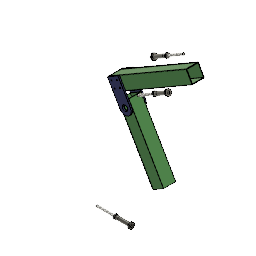
Kerbecs (Autodesk Fusion 360 design; units mm, degrees)
Autodesk Fusion 360 part; units mm, degrees
cylinder "CylinderPrimitive3" add diameter 18 height 736 placed x (0, 0, -1) y (0, 1, 0) z (1, 0, 0) at (0, 0, 0) makes body 1
copy_body "CopyPasteBodies4" bodies 1 makes body 2
move_body "Move2" bodies 2 to x (1, 0, 0) y (0, 1, 0) z (0, 0, 1) at (0, 218, 0)
copy_body "CopyPasteBodies5" bodies 1 2 makes body 3 makes body 4
move_body "Move3" bodies 3 to x (1, 0, 0) y (0, 1, 0) z (0, 0, 1) at (0, 79, 0)
move_body "Move4" bodies 4 to x (1, 0, 0) y (0, 1, 0) z (0, 0, 1) at (0, -79, 0)
cylinder "CylinderPrimitive4" add diameter 18 height 436 placed x (1, 0, 0) y (0, 0, -1) z (0, 1, 0) at (0, 0, 25) separate body makes body 5
move_body "Move5" bodies 5 to x (1, 0, 0) y (0, 1, 0) z (0, 0, 1) at (0, -109, 0)
move_body "Move6" bodies 5 to x (1, 0, 0) y (0, 1, 0) z (0, 0, 1) at (0, 0, -7)
move_body "Move7" bodies 5 to x (1, 0, 0) y (0, 1, 0) z (0, 0, 1) at (9, 0, 0)
copy_body "CopyPasteBodies6" bodies 5 makes body 6
move_body "Move8" bodies 6 to x (1, 0, 0) y (0, 1, 0) z (0, 0, 1) at (318, 0, 0)
copy_body "CopyPasteBodies7" bodies 6 makes body 7
move_body "Move9" bodies 7 to x (1, 0, 0) y (0, 1, 0) z (0, 0, 1) at (132, 0, 0)
copy_body "CopyPasteBodies8" bodies 7 makes body 8
move_body "Move10" bodies 8 to x (1, 0, 0) y (0, 1, 0) z (0, 0, 1) at (318, 0, 0)
move_face "OffsetFaces1" offset 50 1 faces at (736, 0.3267, 5.1676) on bodies 1
move_face "OffsetFaces2" offset 50 1 faces at (736, 79.3267, 5.1676) on bodies 3
move_face "OffsetFaces3" offset 50 1 faces at (736, 141.3455, -1.8705) on bodies 4
move_face "OffsetFaces4" offset 50 1 faces at (736, 220.3455, -1.8705) on bodies 2
move_body "Move11" bodies 5 to x (1, 0, 0) y (0, 1, 0) z (0, 0, 1) at (-18, 0, 0)
move_body "Move12" bodies 5 to x (1, 0, 0) y (0, 1, 0) z (0, 0, 1) at (0, 0, -18)
move_body "Move13" bodies 8 to x (1, 0, 0) y (0, 1, 0) z (0, 0, 1) at (18, 0, -18)
move_body "Move14" bodies 6 7 to x (1, 0, 0) y (0, 1, 0) z (0, 0, 1) at (0, 0, -36)
cylinder "CylinderPrimitive5" add diameter 18 height 200 placed x (1, 0, 0) y (0, 0, -1) z (0, 1, 0) at (0, 0, -75) separate body makes body 9
move_body "Move16" bodies 9 to x (1, 0, 0) y (0, 1, 0) z (0, 0, 1) at (0, -500, 0)
move_body "Move17" bodies 9 to x (1, 0, 0) y (0, 1, 0) z (0, 0, 1) at (0, 0, 75)
move_body "Move18" bodies 9 to x (1, 0, 0) y (0, 0.573576, 0.819152) z (0, -0.819152, 0.573576) at (0, -220.5842, 405.7382)
copy_body "CopyPasteBodies10" bodies 9 makes body 10
move_body "Move19" bodies 10 to x (1, 0, 0) y (0, 1, 0) z (0, 0, 1) at (75, 0, 0)
move_body "Move20" bodies 9 to x (1, 0, 0) y (0, 0.573576, -0.819152) z (0, 0.819152, 0.573576) at (0, -212.1269, -425.492)
move_body "Move21" bodies 10 to x (1, 0, 0) y (0, 0.573576, -0.819152) z (0, 0.819152, 0.573576) at (0, -212.1269, -425.492)
sketch "Sketch8" plane through (0, -506.2875, 0) normal (0, -1, 0) x (1, 0, 0)
  circle A0 centre (0, -12.0782) radius 9
  circle A1 centre (0, -12.0782) radius 9
  line L0 (-13.0767, -7.0782) -> (-23.0767, -7.0782)
  line L1 (-23.0767, -7.0782) -> (-23.0767, -11.0782)
  line L2 (-23.0767, -11.0782) -> (-13.9642, -11.0782)
  line L3 (-13.0767, -17.0782) -> (-23.0767, -17.0782)
  line L4 (-23.0767, -17.0782) -> (-23.0767, -13.0782)
  line L5 (-23.0767, -13.0782) -> (-13.9642, -13.0782)
  arc A2 (-13.0767, -17.0782) -> (13.0767, -17.0782) centre (0, -12.0782) ccw
  arc A3 (13.0767, -7.0782) -> (-13.0767, -7.0782) centre (0, -12.0782) ccw
  line L6 (13.0767, -7.0782) -> (37.5, -7.0782)
  line L7 (13.0767, -17.0782) -> (37.5, -17.0782)
  line L8 (-13.9642, -11.0782) -> (-8.9443, -11.0782)
  line L9 (-13.9642, -13.0782) -> (-8.9443, -13.0782)
  line L10 (98.0767, -11.0782) -> (88.9642, -11.0782)
  line L11 (98.0767, -17.0782) -> (98.0767, -13.0782)
  line L12 (88.0767, -17.0782) -> (98.0767, -17.0782)
  circle A4 centre (75, -12.0782) radius 9
  line L13 (98.0767, -13.0782) -> (88.9642, -13.0782)
  line L14 (61.9233, -17.0782) -> (37.5, -17.0782)
  line L15 (61.9233, -7.0782) -> (37.5, -7.0782)
  arc A5 (88.0767, -7.0782) -> (61.9233, -7.0782) centre (75, -12.0782) ccw
  line L16 (88.0767, -7.0782) -> (98.0767, -7.0782)
  line L17 (88.9642, -13.0782) -> (83.9443, -13.0782)
  arc A6 (61.9233, -17.0782) -> (88.0767, -17.0782) centre (75, -12.0782) ccw
  line L18 (88.9642, -11.0782) -> (83.9443, -11.0782)
  circle A7 centre (75, -12.0782) radius 9
  line L19 (98.0767, -7.0782) -> (98.0767, -11.0782)
  point P0 (75, 0)
  dimension "d85" = 18
  dimension "d86" = 28
  dimension "d90" = 10
  dimension "d91" = 4
  dimension "d92" = 4
  constraint concentric A0 A1
  constraint concentric A1 A2
  constraint coincident A3.start A2
  constraint horizontal L0
  constraint perpendicular L0 L1
  constraint perpendicular L1 L2
  constraint perpendicular L1 L3
  constraint perpendicular L3 L4
  constraint perpendicular L4 L5
  constraint concentric A2 A3
  constraint coincident A1 L8.end
  constraint parallel L2 L8
  constraint coincident A1 L9.end
  constraint parallel L5 L9
  measures "d85" diameter of A1
  measures "d86" diameter of A2
  measures "d90" distance of L0.start L0.end
  measures "d91" distance of L0.end L1.end
  measures "d92" distance of L3.end L4.end
extrude "Extrude4" add sketch "Sketch8" along normal blind 30 separate body contours A0 A1 L0 L1 L2 L3 L4 L5 A2 A3 L6 L7 L8 L9 L10 L11 L12 A4 L13 L14 L15 A5 L16 L17 A6 L18 A7 L19 makes body 11
move_body "Move23" bodies 11 to x (1, 0, 0) y (0, 1, 0) z (0, 0, 1) at (0, -35, 0)
copy_body "CopyPasteBodies11" bodies 11 makes body 12
move_body "Move24" bodies 12 to x (1, 0, 0) y (0, 1, 0) z (0, 0, 1) at (0, -60, 0)
move_body "Move25" bodies 11 to x (1, 0, 0) y (0, 1, 0) z (0, 0, 1) at (0, 230, 0)
move_body "Move26" bodies 12 to x (1, 0, 0) y (0, 1, 0) z (0, 0, 1) at (0, 130, 0)
box "BoxPrimitive1" add length 10 width 215 height 285 placed x (0, 1, 0) y (-1, 0, 0) z (0, 0, 1) at (215, 0, 0) separate body makes body 13
box "BoxPrimitive7" add length 44.45 width 44.45 height 250 placed x (0, 1, 0) y (-1, 0, 0) z (0, 0, 1) at (44.45, 0, 0) separate body makes body 14 in component "Shin"
move_body "Move3'" bodies 14 to x (0.866025, 0, 0.5) y (0, 1, 0) z (-0.5, 0, 0.866025) at (0, 0, 0) in component "Shin"
sketch "Sketch8 (2)" plane through (0, 0, 0) normal (0, -1, 0) x (1, 0, 0) in component "Shin"
  line L0 (-125, 216.5064) -> (0, 0)
  line L1 (0, 0) -> (38.4948, 22.225)
  line L2 (38.4948, 22.225) -> (-86.5052, 238.7314)
  line L3 (-86.5052, 238.7314) -> (-125, 216.5064)
  line L4 (-125, 216.5064) -> (-113.8875, 197.2589)
  line L5 (-113.8875, 197.2589) -> (-94.6401, 208.3714)
  circle A0 centre (-94.6401, 208.3714) radius 9.5
  dimension "d190" = 22.225
  dimension "d191" = 22.225
  dimension "d192" = 19
  constraint coincident L0.start L3.end
  constraint perpendicular L3 L4
  constraint perpendicular L2 L5
  constraint coincident L5.end A0.centre
  measures "d190" distance of L0.start L4.end
  measures "d191" distance of L4.end L5.end
  measures "d192" diameter of A0
hole "Hole1" at (-94.6401, 0, 208.3714) direction (0, 1, 0) diameter 19 depth 44.45 tip angle 180 bodies 14 in component "Shin"
shell "Shell1" thickness 2 removed faces 0 bodies 14 in component "Shin"
sketch "Sketch9" plane through (0, 0, 0) normal (0, -1, 0) x (1, 0, 0) in component "Shin"
  circle A0 centre (-94.6401, 208.3714) radius 9.5
  line L0 (-125, 216.5064) -> (0, 0)
  line L1 (0, 0) -> (38.4948, 22.225)
  line L2 (38.4948, 22.225) -> (-86.5052, 238.7314)
  line L3 (-125, 216.5064) -> (-113.8875, 197.2589)
  line L4 (-75.3927, 219.4839) -> (-86.5052, 238.7314)
  arc A1 (-113.8875, 197.2589) -> (-75.3927, 219.4839) centre (-94.6401, 208.3714) ccw
  line L5 (-125, 216.5064) -> (-149.725, 259.3313)
  line L6 (-86.5052, 238.7314) -> (-111.2302, 281.5563)
  line L7 (-149.725, 259.3313) -> (-111.2302, 281.5563)
  dimension "d199" = 49.45
  constraint coincident L0.start L3.start
  constraint coincident L2.end L4.end
  constraint tangent L3 A1
  constraint tangent L4 A1
  constraint coincident L0 L3.end
  constraint coincident L2 L4.start
  constraint parallel L5 L6
  constraint perpendicular L6 L7
  measures "d199" distance of L0.start L5.end
extrude "Extrude1" add sketch "Sketch9" along normal blind 5 separate body contours L0 L2 L3 L4 A1 L5 L6 L7 makes body 15 in component "Shin"
sketch "Sketch10" plane through (0, -5, 0) normal (0, -1, 0) x (1, 0, 0) in component "Shin"
  circle A0 centre (-94.6401, 208.3714) radius 9.5
  line L0 (-149.725, 259.3313) -> (-113.8875, 197.2589)
  arc A1 (-113.8875, 197.2589) -> (-75.3927, 219.4839) centre (-94.6401, 208.3714) ccw
  line L1 (-75.3927, 219.4839) -> (-111.2302, 281.5563)
  line L2 (-111.2302, 281.5563) -> (-149.725, 259.3313)
  line L3 (-149.725, 259.3313) -> (-144.1687, 249.7076)
  line L4 (-144.1687, 249.7076) -> (-134.545, 255.2638)
  circle A2 centre (-134.545, 255.2638) radius 2
  line L5 (-149.725, 259.3313) -> (-130.4776, 270.4438)
  line L6 (-130.4776, 270.4438) -> (-124.9213, 260.8201)
  line L7 (-149.725, 259.3313) -> (-138.6125, 240.0839)
  line L8 (-138.6125, 240.0839) -> (-100.1177, 262.3089)
  circle A3 centre (-115.2976, 266.3763) radius 2
  circle A4 centre (-123.4325, 236.0164) radius 2
  circle A5 centre (-104.1851, 247.1289) radius 2
  dimension "d206" = 11.1125
  dimension "d207" = 11.1125
  dimension "d208" = 4
  dimension "d212" = 22.225
  constraint coincident L0.start L2.end
  constraint perpendicular L2 L3
  constraint perpendicular L0 L4
  constraint coincident L4.end A2.centre
  constraint midpoint L2 L5.end
  constraint perpendicular L4 L6
  constraint perpendicular L4 L7
  constraint coincident L1 L8.end
  constraint perpendicular L1 L8
  constraint symmetric A2 L6 A3
  constraint symmetric A2 L8 A4
  constraint symmetric L8 A3 A5
  measures "d206" distance of L0.start L3.end
  measures "d207" distance of L3.end L4.end
  measures "d208" diameter of A2
  measures "d212" distance of L0.start L7.end
hole "Hole3" at (-134.545, -5, 255.2638) direction (0, 1, 0) diameter 4 depth 5 tip angle 180 bodies 15 in component "Shin"
hole "Hole2" at (-134.545, -5, 255.2638) direction (0, 1, 0) diameter 4 depth 5 tip angle 180 bodies 15 in component "Shin"
hole "Hole4" at (-115.2976, -5, 266.3763) direction (0, 1, 0) diameter 4 depth 5 tip angle 180 bodies 15 in component "Shin"
hole "Hole5" at (-123.4325, -5, 236.0164) direction (0, 1, 0) diameter 4 depth 5 tip angle 180 bodies 15 in component "Shin"
hole "Hole6" at (-104.1851, -5, 247.1289) direction (0, 1, 0) diameter 4 depth 5 tip angle 180 bodies 15 in component "Shin"
ref_plane "WorkPlane4" through (-109.3509, 22.225, 233.8514) normal (0, 1, 0) x (-1, 0, 0) in component "Shin"
mirror "Mirror1" about plane through (-109.3509, 22.225, 233.8514) normal (0, 1, 0) of bodies 15 makes body 16 in component "Shin"
sketch "Sketch11" plane through (0, 0, 0) normal (0.5, 0, -0.866025) x (0, 1, 0) in component "Shin"
  line L0 (44.45, 0) -> (44.45, 44.45)
  line L1 (44.45, 44.45) -> (0, 44.45)
  line L2 (0, 44.45) -> (0, 0)
  line L3 (0, 0) -> (44.45, 0)
  line L4 (2, 2) -> (42.45, 2)
  line L5 (42.45, 2) -> (42.45, 42.45)
  line L6 (42.45, 42.45) -> (2, 42.45)
  line L7 (2, 42.45) -> (2, 2)
  dimension "d227" = -2
extrude "Extrude2" cut sketch "Sketch11" against normal through all contours L4 L5 L6 L7 bodies 14 in component "Shin"
ref_plane "WorkPlane3" through (-149.725, 44.45, 259.3313) normal (0.866025, 0, 0.5) x (0, 1, 0) in component "Thigh"
sketch "Sketch2" plane through (-149.725, 44.45, 259.3313) normal (0.866025, 0, 0.5) x (0, 1, 0) in component "Thigh"
  line L0 (0, 0) -> (-44.45, 0)
  line L1 (0, 0) -> (0, -44.45)
  dimension "d230" = 44.45
  dimension "d231" = 44.45
  constraint coincident L0.start L1.start
  constraint horizontal L0
  constraint perpendicular L0 L1
  measures "d230" distance of L0.start L0.end
  measures "d231" distance of L0.start L1.end
box "BoxPrimitive1'" add length 44.45 width 44.45 height 320 placed x (0.5, 0, -0.866025) y (0, 1, 0) z (0.866025, 0, 0.5) at (-149.725, 0, 259.3313) separate body makes body 17 in component "Thigh"
sketch "Sketch3" plane through (0, 0, 0) normal (0, -1, 0) x (1, 0, 0) in component "Thigh"
  line L0 (127.4031, 419.3313) -> (-149.725, 259.3313)
  line L1 (-149.725, 259.3313) -> (-127.5, 220.8365)
  line L2 (-127.5, 220.8365) -> (149.6281, 380.8365)
  line L3 (149.6281, 380.8365) -> (127.4031, 419.3313)
  line L4 (-149.725, 259.3313) -> (-144.1687, 249.7076)
  line L5 (-144.1687, 249.7076) -> (-134.545, 255.2638)
  circle A0 centre (-134.545, 255.2638) radius 2
  line L6 (-149.725, 259.3313) -> (-138.6125, 240.0839)
  line L7 (-138.6125, 240.0839) -> (-119.3651, 251.1964)
  line L8 (-119.3651, 251.1964) -> (-130.4776, 270.4438)
  circle A1 centre (-115.2976, 266.3763) radius 2
  circle A2 centre (-104.1851, 247.1289) radius 2
  circle A3 centre (-123.4325, 236.0164) radius 2
  dimension "d237" = 11.1125
  dimension "d238" = 11.1125
  dimension "d239" = 4
  dimension "d241" = 22.225
  dimension "d242" = 22.225
  dimension "d243" = 22.225
  constraint coincident L0.end L1.start
  constraint perpendicular L0 L4
  constraint perpendicular L1 L5
  constraint coincident L5.end A0.centre
  constraint perpendicular L5 L6
  constraint perpendicular L1 L7
  constraint perpendicular L7 L8
  constraint symmetric A0 L8 A1
  constraint symmetric A0 L7 A3
  constraint symmetric L7 A1 A2
  measures "d237" distance of L0.end L4.end
  measures "d238" distance of L4.end L5.end
  measures "d239" diameter of A0
  measures "d241" distance of L0.end L6.end
  measures "d242" distance of L6.end L7.end
  measures "d243" distance of L7.end L8.end
shell "Shell1'" thickness 2 removed faces 1 at (-142.3167, 29.6333, 246.4997) on bodies 17 in component "Thigh"
hole "Hole1'" at (-134.545, 0, 255.2638) direction (0, 1, 0) diameter 4 depth 44.45 tip angle 180 bodies 17 in component "Thigh"
hole "Hole2'" at (-115.2976, 0, 266.3763) direction (0, 1, 0) diameter 4 depth 44.45 tip angle 180 bodies 17 in component "Thigh"
hole "Hole3'" at (-123.4325, 0, 236.0164) direction (0, 1, 0) diameter 4 depth 44.45 tip angle 180 bodies 17 in component "Thigh"
hole "Hole4'" at (-104.1851, 0, 247.1289) direction (0, 1, 0) diameter 4 depth 44.45 tip angle 180 bodies 17 in component "Thigh"
delete_face "DeleteFace1" 1 faces at (133.4127, 28.9667, 404.9223) on bodies 17 in component "Thigh"
move_face "OffsetFaces1'" offset 17.225 2 faces at (-136.8934, -1.6667, 266.7396) (-136.8934, 46.1167, 266.7396) on bodies 15 16 in component "Shin"
move_face "MoveFace1" to x (1, 0, 0) y (0, 1, 0) z (0, 0, 1) at (-8.6125, 0, 14.9173) 8 faces at (-115.9817, -3.3333, 264.497) (-135.0386, -3.3333, 257.202) (-104.8692, -3.3333, 245.2496) (-124.1166, -3.3333, 234.1371) (-115.9817, 47.7833, 268.2557) (-134.0515, 47.7833, 257.202) (-124.1166, 47.7833, 237.8958) (-104.8692, 47.7833, 249.0083) on bodies 15 16 in component "Shin"
copy_body "Body->Comp1" bodies 14 removing the originals makes body 18 in component "Bone"
copy_body "Body->Comp2" bodies 16 removing the originals makes body 19 in component "Component"
copy_body "Body->Comp3" bodies 15 removing the originals makes body 20 in component "Component'"
cylinder "CylinderPrimitive1" add diameter 8 height 100 placed x (0, 0, -1) y (0, 1, 0) z (1, 0, 0) at (0, -200, 50) separate body makes body 21 in component "Component''"
thread "Thread1" "ISO Metric profile 8.0 M8x1.25 6g" major diameter 7.866 minor diameter 6.4455 pitch 1.25 angle 60 resizes the face on face at (33.3333, -198.087, 53.5129) on bodies 21 in component "Component''"
cylinder "CylinderPrimitive1'" add diameter 15 height 5 placed x (0, 0, -1) y (0, 1, 0) z (1, 0, 0) at (100, -200, 50) separate body makes body 22 in component "Component'''"
hole "Hole1''" at (105, -200, 50) direction (-1, 0, 0) diameter 8 end up to surface (5 mm away) bodies 22 in component "Component'''"
sketch "Sketch10 (2)" plane through (70, 0, 0) normal (1, 0, 0) x (0, 1, 0)
  circle A0 centre (-200, 50) radius 4
  circle A1 centre (-200, 50) radius 7.5
  circle A2 centre (-200, 50) radius 5
  dimension "d291" = 10
  constraint concentric A0 A2
  measures "d291" diameter of A2
extrude "Extrude1'" add sketch "Sketch10 (2)" along normal blind 10 contours A2 sketch seen with x (1, 0, 0) y (0, 1, 0) z (0, 0, 1) at (35, 0, 0) bodies 22 in component "Component'''"
ref_plane "WorkPlane1" through (80, -200, 50) normal (1, 0, 0) x (0, 1, 0) in component "Component''''"
cylinder "CylinderPrimitive1''" add diameter 13 height 50 placed x (0, 0, -1) y (0, 1, 0) z (1, 0, 0) at (80, -200, 50) separate body makes body 23 in component "Component''''"
hole "Hole1'''" at (130, -200, 50) direction (-1, 0, 0) diameter 10 depth 50 tip angle 180 bodies 21 in component "Component''"
hole "Hole1''''" at (130, -200, 50) direction (-1, 0, 0) diameter 10 depth 50 tip angle 180 bodies 23 in component "Component''''"
sketch "Sketch2 (2)" plane through (130, 0, 0) normal (1, 0, 0) x (0, 1, 0) in component "Component''''"
  circle A0 centre (-200, 50) radius 5
  circle A1 centre (-200, 50) radius 6.5
  line L0 (-200, 50) -> (-190, 50)
  circle A2 centre (-200, 50) radius 10
  dimension "d303" = 10
  constraint coincident A0.centre A1.centre
  constraint horizontal L0
  constraint coincident L0.end A2
  measures "d303" distance of A0.centre L0.end
extrude "Extrude1''" add sketch "Sketch2 (2)" along normal blind 5 contours A1 | A2 bodies 23 in component "Component''''"
cylinderprimitive "CylinderPrimitive2" [suppressed]
component "Shin" placed x (1, 0, 0) y (0, 1, 0) z (0, 0, 1) at (-8.6125, 0, 14.9173)
component "Thigh" placed x (1, 0, 0) y (0, 1, 0) z (0, 0, 1) at (-8.6125, 0, 14.9173)
component "Component''" placed x (1, 0, 0) y (0, 1, 0) z (0, 0, 1) at (0, 0, 0)
component "Component'''" placed x (1, 0, 0) y (0, 1, 0) z (0, 0, 1) at (-35, 0, 0)
component "Component''''" placed x (1, 0, 0) y (0, 1, 0) z (0, 0, 1) at (-10, 0, 0)
component "Component''" placed x (0.866025, 0, 0.5) y (0, 1, 0) z (-0.5, 0, 0.866025) at (-17.1891, 225, 219.0544)
component "Component'''" placed x (0.866025, 0, 0.5) y (0, 1, 0) z (-0.5, 0, 0.866025) at (-47.5, 225, 201.5544)
component "Component''''" placed x (0.866025, 0, 0.5) y (0, 1, 0) z (-0.5, 0, 0.866025) at (-25.8494, 225, 214.0544)
component "Component''" placed x (0.866025, 0, 0.5) y (0, 1, 0) z (-0.5, 0, 0.866025) at (-17.1891, 225, 219.0544)
component "Component'''" placed x (0.866025, 0, 0.5) y (0, 1, 0) z (-0.5, 0, 0.866025) at (-47.5, 225, 201.5544)
component "Component''''" placed x (0.866025, 0, 0.5) y (0, 1, 0) z (-0.5, 0, 0.866025) at (-25.8494, 225, 214.0544)
component "Bone" placed x (1, 0, 0) y (0, 1, 0) z (0, 0, 1) at (8.6125, 0, -14.9173) in component "Shin"
component "Component" placed x (1, 0, 0) y (0, 1, 0) z (0, 0, 1) at (8.6125, 0, -14.9173) in component "Shin"
component "Component'" placed x (1, 0, 0) y (0, 1, 0) z (0, 0, 1) at (8.6125, 0, -14.9173) in component "Shin"
equation "d11 = 18.00 mm + 200 mm"
equation "d14 = ( ( 18 + 200 ) / 2 ) * 1 mm - 30 mm"
equation "d17 = -( ( ( 18 + 200 ) / 2 ) * 1 mm - 30 mm )"
equation "d33 = 114 mm + 18 mm"
equation "d190 = ( 44.45 / 2 ) * 1 mm"
equation "d191 = ( 44.450 / 2 ) * 1 mm"
equation "d199 = 44.45 mm + 5 mm"
equation "d206 = ( 44.45 / 4 ) * 1 mm"
equation "d207 = ( 44.45 / 4 ) * 1 mm"
equation "d212 = ( 44.45 / 2 ) * 1 mm"
equation "d225 = ( 44.45 / 2 ) * 1 mm"
equation "d237 = ( 44.45 / 4 ) * 1 mm"
equation "d241 = ( 44.45 / 2 ) * 1 mm"
equation "d242 = ( 44.45 / 2 ) * 1 mm"
equation "d243 = ( 44.45 / 2 ) * 1 mm"
equation "d257 = ( ( 44.45 / 2 ) * 1 mm ) - 5 mm"
equation "d258 = ( ( 44.45 / 2 ) * 1 mm ) - 5 mm"
named bodies: "Pipe 1", "Pipe 4", "Pipe 1 (1)", "Pipe 1 (1) (1)", "Pipe 2", "Pipe 3", "Pipe 5", "Pipe 6", "Pipe 5 (1)", "Pipe 7", "Pipe 5 (1) (1)", "Pipe8", "Thigh 1", "Thigh 2", "Thigh Clamp 1", "Thigh Clamp 2"
